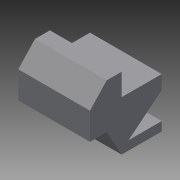
# Autodesk Inventor part: 136
Saved by Autodesk Inventor 2014 (Build 180170000, 170)
## iProperties
Created: 2017-04-22
Part Number: 136
Material: Generic
Document SubType Name: Modeling
Designer: Andy
Density: 1 g/cm^3
Appearance: Default
Author: Andy
Autodesk Inventor part; units mm, degrees
ref_plane "YZ Plane" through (0, 0, 0) normal (1, 0, 0) x (0, 1, 0)
ref_plane "XZ Plane" through (0, 0, 0) normal (0, 1, 0) x (-1, 0, 0)
ref_plane "XY Plane" through (0, 0, 0) normal (0, 0, 1) x (1, 0, 0)
sketch "Sketch3" plane through (0, 0, 0) normal (0, 1, 0) x (-1, 0, 0)
  line L0 (0, 0) -> (10, 0)
  line L1 (10, 0) -> (10, -10)
  line L2 (10, -10) -> (0, -10)
  line L3 (0, -10) -> (0, 0)
  dimension "d7" = 10
  dimension "d8" = 10
  constraints: 8 end point, 2 parallel, 1 horizontal, 1 perpendicular
  measures "d7" distance of L1.end L2.end
  measures "d8" distance of L0.end L1.end
extrude "Extrusion1" add sketch "Sketch3" along normal blind 10
sketch "Sketch4" plane through (0, 0, 0) normal (1, 0, 0) x (0, 0, -1)
  line L0 (10, 0) -> (0, 0) projected
  line L1 (0, 0) -> (0, 10) projected
  line L2 (0, 0) -> (2.5, 0)
  line L3 (2.5, 0) -> (0, 2.3259)
  dimension "d11" = 2.5
  constraints: 4 end point, 2 point on line
  measures "d11" distance of L0.end L2.end
extrude "Extrusion2" cut sketch "Sketch4" against normal blind 10
sketch "Sketch5" plane through (0, 0, -10) normal (1, 0, 0) x (0, 0, -1)
  line L0 (0, 0) -> (-7.5, 0) projected
  line L1 (0, 0) -> (0, 10) projected
  line L2 (-10, 10) -> (0, 10) projected
  line L3 (-10, 2.3259) -> (-10, 10) projected
  line L4 (-3.75, 0) -> (-3.75, 2.3259)
  line L5 (-3.75, 2.3259) -> (0, 4.4117)
  line L6 (0, 0) -> (-3.75, 0)
  line L7 (-1.5, 10) -> (-1.5, 6)
  line L8 (-1.5, 6) -> (-4.6791, 10)
  point P0 (-10, 0)
  dimension "d14" = 4
  constraints: 10 end point, 3 point on line, 2 perpendicular, 1 midpoint, 1 parallel
  measures "d14" distance of L7.start L7.end
extrude "Extrusion3" cut sketch "Sketch5" against normal blind 10 contours L0 L4 L5 L1
sketch "Sketch6" plane through (0, 10, 0) normal (1, 0, 0) x (0, 0, -1)
  line L0 (0, 0) -> (10, 0) projected
  line L1 (6.25, -10) -> (2.5, -10) projected
  line L2 (8.75, 0) -> (8.75, -4.6256)
  line L3 (8.75, -4.6256) -> (5, 0)
  line L4 (5, 0) -> (8.75, 0)
  point P0 (0, -10)
  constraints: 6 end point, 2 perpendicular, 1 midpoint, 1 point on line
extrude "Extrusion4" cut sketch "Sketch6" against normal blind 10
sketch "Sketch7" plane through (0, 2.3259, 0) normal (1, 0, 0) x (0, 0, -1)
  line L0 (0, 7.6741) -> (5, 7.6741) projected
  line L1 (0, 0) -> (0, 7.6741) projected
  line L2 (3.0747, 7.6741) -> (0, 7.6741)
  line L3 (0, 7.6741) -> (0, 2.0858)
  line L4 (0, 2.0858) -> (3.0747, 2.0858)
  line L5 (3.0747, 2.0858) -> (3.0747, 7.6741)
  point P0 (0, -2.3259)
  constraints: 8 end point, 2 parallel, 2 point on line, 1 horizontal, 1 perpendicular
extrude "Extrusion5" cut sketch "Sketch7" against normal blind 10
body "Solid1"
